Autodesk Inventor part; units mm, degrees
(part 2 of 2)
  spline S168 degree 2 poles (30.2962, -217.2786) (29.7923, -217.2786) (29.3205, -216.4956) (29.3205, -215.6929) knots 0 0 0 1 2 2 2
  spline S169 degree 2 poles (29.3205, -215.6929) (29.3205, -214.8679) (29.7972, -214.1047) (30.2962, -214.1047) knots 0 0 0 1 2 2 2
  spline S170 degree 2 poles (30.2962, -214.1047) (30.7976, -214.1047) (31.2693, -214.8951) (31.2693, -215.6904) knots 0 0 0 1 2 2 2
  spline S171 degree 2 poles (30.7457, -216.6191) (30.805, -216.4685) (30.8544, -216.0041) (30.8544, -215.6904) knots 0 0 0 1 2 2 2
  spline S172 degree 2 poles (30.8544, -215.6904) (30.8544, -215.3767) (30.805, -214.9148) (30.7432, -214.7592) knots 0 0 0 1 2 2 2
  spline S173 degree 2 poles (30.7432, -214.7592) (30.6815, -214.6036) (30.4666, -214.4431) (30.2962, -214.4431) knots 0 0 0 1 2 2 2
  spline S174 degree 2 poles (30.2962, -214.4431) (30.1257, -214.4431) (29.9059, -214.6036) (29.8417, -214.7642) knots 0 0 0 1 2 2 2
  spline S175 degree 2 poles (29.8417, -214.7642) (29.7799, -214.9198) (29.7355, -215.394) (29.7355, -215.6929) knots 0 0 0 1 2 2 2
  spline S176 degree 2 poles (29.7355, -215.6929) (29.7355, -216.014) (29.775, -216.4438) (29.8392, -216.6117) knots 0 0 0 1 2 2 2
  spline S177 degree 2 poles (29.8392, -216.6117) (29.8985, -216.7698) (30.1183, -216.9402) (30.2962, -216.9402) knots 0 0 0 1 2 2 2
  spline S178 degree 2 poles (30.2962, -216.9402) (30.4641, -216.9402) (30.684, -216.7797) (30.7457, -216.6191) knots 0 0 0 1 2 2 2
  line L158 (33.5393, -217.2144) -> (31.6596, -217.2144)
  line L159 (31.6596, -217.2144) -> (31.6596, -216.7822)
  spline S179 degree 2 poles (31.6596, -216.7822) (31.8622, -216.592) (32.2228, -216.2388) (32.3957, -216.0486) knots 0 0 0 1 2 2 2
  spline S180 degree 2 poles (32.3957, -216.0486) (32.7439, -215.6657) (32.9984, -215.2063) (32.9984, -214.9618) knots 0 0 0 1 2 2 2
  spline S181 degree 2 poles (32.9984, -214.9618) (32.9984, -214.8333) (32.9193, -214.6407) (32.8477, -214.5789) knots 0 0 0 1 2 2 2
  spline S182 degree 2 poles (32.8477, -214.5789) (32.7761, -214.5172) (32.5883, -214.4554) (32.4747, -214.4554) knots 0 0 0 1 2 2 2
  spline S183 degree 2 poles (32.4747, -214.4554) (32.366, -214.4554) (32.1437, -214.5097) (32.0425, -214.5517) knots 0 0 0 1 2 2 2
  spline S184 degree 2 poles (32.0425, -214.5517) (31.956, -214.5863) (31.7955, -214.6851) (31.7461, -214.7197) knots 0 0 0 1 2 2 2
  line L160 (31.7461, -214.7197) -> (31.7238, -214.7197)
  line L161 (31.7238, -214.7197) -> (31.7238, -214.285)
  spline S185 degree 2 poles (31.7238, -214.285) (31.8498, -214.2232) (32.3018, -214.1022) (32.5044, -214.1022) knots 0 0 0 1 2 2 2
  spline S186 degree 2 poles (32.5044, -214.1022) (32.9317, -214.1022) (33.4133, -214.5542) (33.4133, -214.9395) knots 0 0 0 1 2 2 2
  spline S187 degree 2 poles (33.4133, -214.9395) (33.4133, -215.1198) (33.3293, -215.4212) (33.2552, -215.5496) knots 0 0 0 1 2 2 2
  spline S188 degree 2 poles (33.2552, -215.5496) (33.1811, -215.683) (32.9663, -215.9448) (32.8477, -216.0708) knots 0 0 0 1 2 2 2
  spline S189 degree 2 poles (32.8477, -216.0708) (32.655, -216.2807) (32.1833, -216.7303) (32.0425, -216.8612) knots 0 0 0 1 2 2 2
  line L162 (32.0425, -216.8612) -> (33.5393, -216.8612)
  line L163 (33.5393, -216.8612) -> (33.5393, -217.2144)
  spline S190 degree 2 poles (35.8735, -216.2264) (35.8735, -216.4611) (35.7178, -216.8587) (35.5869, -216.9921) knots 0 0 0 1 2 2 2
  spline S191 degree 2 poles (35.5869, -216.9921) (35.4511, -217.1329) (35.1102, -217.2786) (34.9052, -217.2786) knots 0 0 0 1 2 2 2
  spline S192 degree 2 poles (34.9052, -217.2786) (34.7002, -217.2786) (34.3618, -217.1403) (34.2334, -217.002) knots 0 0 0 1 2 2 2
  spline S193 degree 2 poles (34.2334, -217.002) (34.0753, -216.8365) (33.8974, -216.2807) (33.8974, -215.8757) knots 0 0 0 1 2 2 2
  spline S194 degree 2 poles (33.8974, -215.8757) (33.8974, -215.478) (34.0605, -214.8383) (34.2309, -214.6011) knots 0 0 0 1 2 2 2
  spline S195 degree 2 poles (34.2309, -214.6011) (34.3964, -214.369) (34.92, -214.1096) (35.2634, -214.1096) knots 0 0 0 1 2 2 2
  spline S196 degree 2 poles (35.2634, -214.1096) (35.3646, -214.1096) (35.5425, -214.1294) (35.6092, -214.1516) knots 0 0 0 1 2 2 2
  line L164 (35.6092, -214.1516) -> (35.6092, -214.5443)
  line L165 (35.6092, -214.5443) -> (35.5919, -214.5443)
  spline S197 degree 2 poles (35.5919, -214.5443) (35.5351, -214.5147) (35.3276, -214.4628) (35.209, -214.4628) knots 0 0 0 1 2 2 2
  spline S198 degree 2 poles (35.209, -214.4628) (34.8286, -214.4628) (34.3618, -214.9766) (34.3173, -215.4805) knots 0 0 0 1 2 2 2
  spline S199 degree 2 poles (34.3173, -215.4805) (34.4631, -215.3792) (34.7694, -215.268) (34.9521, -215.268) knots 0 0 0 1 2 2 2
  spline S200 degree 2 poles (34.9521, -215.268) (35.13, -215.268) (35.3967, -215.3397) (35.5425, -215.4484) knots 0 0 0 1 2 2 2
  spline S201 degree 2 poles (35.5425, -215.4484) (35.7104, -215.5743) (35.8735, -215.9646) (35.8735, -216.2264) knots 0 0 0 1 2 2 2
  spline S202 degree 2 poles (35.4585, -216.2437) (35.4585, -216.056) (35.3597, -215.8016) (35.251, -215.7126) knots 0 0 0 1 2 2 2
  spline S203 degree 2 poles (35.251, -215.7126) (35.1695, -215.6484) (34.967, -215.6064) (34.8608, -215.6064) knots 0 0 0 1 2 2 2
  spline S204 degree 2 poles (34.8608, -215.6064) (34.7175, -215.6064) (34.4483, -215.6929) (34.3173, -215.7744) knots 0 0 0 1 2 2 2
  spline S205 degree 2 poles (34.3173, -215.7744) (34.3149, -215.8189) (34.3099, -215.9028) (34.3099, -215.9671) knots 0 0 0 1 2 2 2
  spline S206 degree 2 poles (34.3099, -215.9671) (34.3099, -216.2832) (34.4334, -216.671) (34.5273, -216.7723) knots 0 0 0 1 2 2 2
  spline S207 degree 2 poles (34.5273, -216.7723) (34.6138, -216.8686) (34.8015, -216.9452) (34.9077, -216.9452) knots 0 0 0 1 2 2 2
  spline S208 degree 2 poles (34.9077, -216.9452) (35.1547, -216.9452) (35.4585, -216.5944) (35.4585, -216.2437) knots 0 0 0 1 2 2 2
  point P0 (0, 0)
  constraints: 2 other
emboss "Emboss1" sketch "Sketch14" operation cut depth 2.54 direction (-1, 0, 0)
sketch "Sketch16" plane through (5.08, 0, 0) normal (1, 0, 0) x (0, 0, -1)
  line L0 (-41.7074, -88.6682) -> (39.5726, -88.6682)
  line L1 (39.5726, -88.6682) -> (39.5726, -92.4782)
  line L2 (39.5726, -92.4782) -> (-41.7074, -92.4782)
  line L3 (-41.7074, -92.4782) -> (-41.7074, -88.6682)
  line L4 (22.7938, -210.0802) -> (-43.6417, -210.0802) projected
  line L5 (38.9083, -223.7962) -> (-43.6417, -223.7962) projected
  point P0 (0, 0)
  dimension "d195" = 3.81
  dimension "d692" = 135.128
  constraints: 8 end point, 2 parallel, 1 horizontal, 1 perpendicular
  measures "d195" distance between parallel lines of L0 L2
  measures "d692" distance between parallel lines of L5 L0
extrude "Extrusion13" add sketch "Sketch16" along normal blind 5.08
sketch "Sketch17" plane through (22.86, 33.2264, 21.4167) normal (0, 1, 0) x (1, 0, 0)
  line L0 (-6.858, 38.1) -> (0, 38.1) projected
  line L1 (-0.0061, 38.1) -> (0.0392, 38.1)
  line L2 (0, 65.5066) -> (0, -27.4066) projected
  line L3 (0, 35.5801) -> (0, 35.5243)
  line L4 (5, -24.2316) -> (5, 62.3316) projected
  line L5 (0, 38.1) -> (5, 38.1)
  line L6 (5, 38.1) -> (5, 0)
  line L7 (5, 0) -> (0, 0)
  line L8 (0, 0) -> (0, 38.1)
  point P0 (-22.86, 21.4167)
  point P1 (5, -23.8506)
  point P2 (5, 69.0626)
  point P3 (0, 0)
  point P4 (5, 38.1)
  point P5 (0, 38.1)
  point P6 (2.5, 0)
  point P7 (2.5, 38.1)
  dimension "d689" = 38.1
  constraints: 12 end point, 4 point on line, 2 horizontal, 2 midpoint, 2 parallel, 1 perpendicular
  measures "d689" distance of point (2.5, 0) point (2.5, 38.1)
extrude "Extrusion14" cut sketch "Sketch17" against normal blind 2.0066
sketch "Sketch18" plane through (0, 0, 0) normal (-1, 0, 0) x (0, 0, 1)
  arc A0 (46.2144, 33.1755) -> (48.7724, 30.6175) centre (48.0867, 32.4898) ccw projected
  circle A1 centre (48.0867, 32.4898) radius 4.5085
  arc A2 (-41.481, 33.1755) -> (-44.039, 30.6175) centre (-43.3533, 32.4898) ccw projected
  circle A3 centre (-43.3533, 32.4898) radius 4.5085
  arc A4 (-44.039, -223.194) -> (-41.481, -225.752) centre (-43.3533, -225.0662) ccw projected
  circle A5 centre (-43.3533, -225.0662) radius 4.5085
  arc A6 (46.2144, -225.752) -> (48.7724, -223.194) centre (48.0867, -225.0662) ccw projected
  circle A7 centre (48.0867, -225.0662) radius 4.5085
  point P0 (0, 0)
  dimension "d209" = 9.017
  dimension "d210" = 9.017
  dimension "d211" = 9.017
  dimension "d212" = 9.017
  constraints: 4 centre point, 4 coincident
  measures "d209" diameter of A1
  measures "d210" diameter of A3
  measures "d211" diameter of A5
  measures "d212" diameter of A7
extrude "Extrusion15" [suppressed]
sketch "Sketch19" plane through (22.86, -64.2842, -44.0899) normal (0, 0, -1) x (-1, 0, 0)
  line L0 (6.35, 0) -> (0, 0) projected
  line L1 (-5, 92.329) -> (-5, -156.337) projected
  line L2 (0, 0) -> (-5, 0)
  line L3 (-5, 0) -> (-5, 8.001)
  line L4 (-5, 8.001) -> (0, 8.001)
  line L5 (0, 8.001) -> (0, 0)
  point P0 (22.86, 64.2842)
  dimension "d216" = 5
  dimension "d219" = 8.001
  constraints: 8 end point, 2 parallel, 1 horizontal, 1 perpendicular, 1 point on line
  measures "d216" distance between parallel lines of L1 L5
  measures "d219" distance between parallel lines of L2 L4
extrude "Extrusion16" cut sketch "Sketch19" against normal blind 24.13
sketch "Sketch20" plane through (0, 0, 0) normal (-1, 0, 0) x (0, 0, 1)
  line L0 (-45.1249, 28.9592) -> (-41.5943, 28.9592)
  line L1 (-45.1249, 36.0204) -> (-41.5943, 36.0204)
  line L2 (-45.1249, 28.9592) -> (-47.1633, 32.4898)
  line L3 (-45.1249, 36.0204) -> (-47.1633, 32.4898)
  line L4 (-41.5943, 28.9592) -> (-39.5559, 32.4898)
  line L5 (-41.5943, 36.0204) -> (-39.5559, 32.4898)
  line L6 (49.8457, 36.0204) -> (51.8841, 32.4898)
  line L7 (49.8457, 28.9592) -> (51.8841, 32.4898)
  line L8 (46.3151, 28.9592) -> (49.8457, 28.9592)
  line L9 (46.3151, 36.0204) -> (49.8457, 36.0204)
  line L10 (46.3151, 36.0204) -> (44.2767, 32.4898)
  line L11 (46.3151, 28.9592) -> (44.2767, 32.4898)
  line L12 (-41.5943, -210.3596) -> (-39.5559, -213.8902)
  line L13 (-41.5943, -217.4208) -> (-39.5559, -213.8902)
  line L14 (-45.1249, -217.4208) -> (-41.5943, -217.4208)
  line L15 (-45.1249, -210.3596) -> (-41.5943, -210.3596)
  line L16 (-45.1249, -210.3596) -> (-47.1633, -213.8902)
  line L17 (-45.1249, -217.4208) -> (-47.1633, -213.8902)
  line L18 (49.8457, -210.3596) -> (51.8841, -213.8902)
  line L19 (49.8457, -217.4208) -> (51.8841, -213.8902)
  line L20 (46.3151, -217.4208) -> (49.8457, -217.4208)
  line L21 (46.3151, -210.3596) -> (49.8457, -210.3596)
  line L22 (46.3151, -210.3596) -> (44.2767, -213.8902)
  line L23 (46.3151, -217.4208) -> (44.2767, -213.8902)
  line L24 (43.6417, 31.2198) -> (-38.9083, 31.2198) projected
  line L25 (-45.2583, 37.5698) -> (49.9917, 37.5698) projected
  line L26 (53.1667, 34.3948) -> (53.1667, -226.9712) projected
  line L27 (41.2351, -73.1996) -> (44.7657, -73.1996)
  line L28 (44.7657, -73.1996) -> (46.8041, -76.7302)
  line L29 (41.2351, -73.1996) -> (39.1967, -76.7302)
  line L30 (44.7657, -80.2608) -> (46.8041, -76.7302)
  line L31 (41.2351, -80.2608) -> (39.1967, -76.7302)
  line L32 (41.2351, -80.2608) -> (44.7657, -80.2608)
  line L33 (-40.0449, -73.1996) -> (-42.0833, -76.7302)
  line L34 (-40.0449, -80.2608) -> (-42.0833, -76.7302)
  line L35 (-40.0449, -73.1996) -> (-36.5143, -73.1996)
  line L36 (-40.0449, -80.2608) -> (-36.5143, -80.2608)
  line L37 (-36.5143, -73.1996) -> (-34.4759, -76.7302)
  line L38 (-36.5143, -80.2608) -> (-34.4759, -76.7302)
  line L39 (-48.4333, -226.9712) -> (-48.4333, 34.3948) projected
  point P0 (0, 0)
  point P1 (-43.3596, 28.9592)
  point P2 (-43.3533, 32.4898)
  point P3 (48.0804, 28.9592)
  point P4 (-43.3596, -217.4208)
  point P5 (48.0804, -217.4208)
  point P6 (-16.6833, 31.2198)
  point P7 (43.0004, -80.2608)
  point P8 (-38.2796, -80.2608)
  dimension "d366" = 7.0612
  dimension "d367" = 120
  dimension "d368" = 120
  dimension "d369" = 120
  dimension "d370" = 120
  dimension "d371" = 3.5306
  dimension "d372" = 3.5306
  dimension "d373" = 3.5306
  dimension "d374" = 3.5306
  dimension "d375" = 3.5306
  dimension "d376" = 3.5306
  dimension "d377" = 0
  dimension "d378" = 7.6074
  dimension "d383" = 7.0612
  dimension "d384" = 120
  dimension "d385" = 120
  dimension "d386" = 120
  dimension "d387" = 120
  dimension "d388" = 3.5306
  dimension "d389" = 3.5306
  dimension "d390" = 3.5306
  dimension "d391" = 3.5306
  dimension "d392" = 3.5306
  dimension "d393" = 3.5306
  dimension "d394" = 0
  dimension "d395" = 7.6074
  dimension "d402" = 7.0612
  dimension "d403" = 120
  dimension "d404" = 120
  dimension "d405" = 120
  dimension "d406" = 120
  dimension "d407" = 3.5306
  dimension "d408" = 3.5306
  dimension "d409" = 3.5306
  dimension "d410" = 3.5306
  dimension "d411" = 3.5306
  dimension "d412" = 3.5306
  dimension "d413" = 0
  dimension "d414" = 7.6074
  dimension "d421" = 7.0612
  dimension "d422" = 120
  dimension "d423" = 120
  dimension "d424" = 120
  dimension "d425" = 120
  dimension "d426" = 3.5306
  dimension "d427" = 3.5306
  dimension "d428" = 3.5306
  dimension "d429" = 3.5306
  dimension "d430" = 3.5306
  dimension "d431" = 3.5306
  dimension "d432" = 0
  dimension "d433" = 7.6074
  dimension "d731" = 7.0612
  dimension "d732" = 120
  dimension "d733" = 120
  dimension "d734" = 120
  dimension "d735" = 120
  dimension "d736" = 3.5306
  dimension "d737" = 3.5306
  dimension "d738" = 3.5306
  dimension "d739" = 3.5306
  dimension "d740" = 3.5306
  dimension "d741" = 3.5306
  dimension "d742" = 0
  constraints: 72 end point, 12 horizontal, 6 midpoint
  measures "d366" distance from line of point (-43.36, 28.959) L1
  measures "d367" angle of L0 L2
  measures "d368" angle of L1 L3
  measures "d369" angle of L4 L0
  measures "d370" angle of L5 L1
  measures "d371" distance of L0.start L4.start
  measures "d372" distance of L1.start L5.start
  measures "d373" vertical distance of L1.start L3.end
  measures "d374" vertical distance of L0.start L2.end
  measures "d375" vertical distance of L5.start L5.end
  measures "d376" vertical distance of L4.start L4.end
  measures "d377" horizontal distance of L0.start L1.start
  measures "d378" distance of L4.end L2.end
  measures "d383" distance from line of point (48.08, 28.959) L9
  measures "d384" angle of L8 L11
  measures "d385" angle of L9 L10
  measures "d386" angle of L7 L8
  measures "d387" angle of L6 L9
  measures "d388" distance of L8.start L7.start
  measures "d389" distance of L9.start L6.start
  measures "d390" vertical distance of L9.start L10.end
  measures "d391" vertical distance of L8.start L11.end
  measures "d392" vertical distance of L6.start L6.end
  measures "d393" vertical distance of L7.start L7.end
  measures "d394" horizontal distance of L8.start L9.start
  measures "d395" distance of L7.end L11.end
  measures "d402" distance from line of point (-43.36, -217.421) L15
  measures "d403" angle of L14 L17
  measures "d404" angle of L15 L16
  measures "d405" angle of L13 L14
  measures "d406" angle of L12 L15
  measures "d407" distance of L14.start L13.start
  measures "d408" distance of L15.start L12.start
  measures "d409" vertical distance of L15.start L16.end
  measures "d410" vertical distance of L14.start L17.end
  measures "d411" vertical distance of L12.start L12.end
  measures "d412" vertical distance of L13.start L13.end
  measures "d413" horizontal distance of L14.start L15.start
  measures "d414" distance of L13.end L17.end
  measures "d421" distance from line of point (48.08, -217.421) L21
  measures "d422" angle of L20 L23
  measures "d423" angle of L21 L22
  measures "d424" angle of L19 L20
  measures "d425" angle of L18 L21
  measures "d426" distance of L20.start L19.start
  measures "d427" distance of L21.start L18.start
  measures "d428" vertical distance of L21.start L22.end
  measures "d429" vertical distance of L20.start L23.end
  measures "d430" vertical distance of L18.start L18.end
  measures "d431" vertical distance of L19.start L19.end
  measures "d432" horizontal distance of L20.start L21.start
  measures "d433" distance of L19.end L23.end
  measures "d731" distance from line of point (43, -80.261) L27
  measures "d732" angle of L32 L31
  measures "d733" angle of L27 L29
  measures "d734" angle of L30 L32
  measures "d735" angle of L28 L27
  measures "d736" distance of L31.start L32.end
  measures "d737" distance of L29.start L27.end
  measures "d738" vertical distance of L29.start L29.end
  measures "d739" vertical distance of L31.start L31.end
  measures "d740" vertical distance of L27.end L28.end
  measures "d741" vertical distance of L32.end L30.end
  measures "d742" horizontal distance of L31.start L29.start
extrude "Extrusion18" cut sketch "Sketch20" against normal blind 4
sketch "Sketch21" plane through (5.08, 0, 0) normal (1, 0, 0) x (0, 0, -1)
  line L0 (-46.8167, -220.6212) -> (-46.8167, 28.0448) projected
  line L1 (35.2253, -82.5002) -> (35.2253, -72.3775)
  line L2 (42.0833, -65.4455) -> (42.0833, -88.8822)
  circle A0 centre (38.2733, -76.7302) radius 1.9939
  line L3 (42.0833, -69.6717) -> (42.0833, -83.8957)
  line L4 (35.2282, -81.9518) -> (35.2282, -71.6157)
  line L5 (36.9596, -68.7879) -> (40.1092, -67.18)
  line L6 (41.4701, -65.8406) -> (42.0833, -64.6853)
  line L7 (36.9596, -84.7796) -> (40.1092, -86.3875)
  line L8 (41.4701, -87.7269) -> (42.0833, -88.8822)
  arc A1 (36.9596, -68.7879) -> (35.2282, -71.6157) centre (38.4032, -71.6157) ccw
  arc A2 (40.1092, -67.18) -> (41.4701, -65.8406) centre (38.6656, -64.3522) ccw
  arc A3 (35.2282, -81.9518) -> (36.9596, -84.7796) centre (38.4032, -81.9518) ccw
  arc A4 (41.4701, -87.7269) -> (40.1092, -86.3875) centre (38.6656, -89.2153) ccw
  circle A5 centre (38.2733, -76.7302) radius 1.9939 projected
  line L9 (44.0899, -222.6278) -> (44.0899, -64.2842) projected
  line L10 (42.0833, -65.4455) -> (42.0833, -64.6853)
  line L11 (-46.8167, -83.8422) -> (-46.8167, -69.6182)
  line L12 (-39.9587, -71.5622) -> (-39.9587, -81.8983)
  circle A6 centre (-43.0067, -76.7302) radius 1.9939 projected
  line L13 (-41.6901, -84.7261) -> (-44.8397, -86.334)
  line L14 (-46.1908, -87.655) -> (-46.8167, -88.8159)
  line L15 (-41.6901, -68.7344) -> (-44.8397, -67.1265)
  line L16 (-46.2239, -65.7423) -> (-46.8167, -64.5811)
  arc A7 (-44.8397, -86.334) -> (-46.1908, -87.655) centre (-43.3961, -89.1618) ccw
  arc A8 (-41.6901, -84.7261) -> (-39.9587, -81.8983) centre (-43.1337, -81.8983) ccw
  arc A9 (-39.9587, -71.5622) -> (-41.6901, -68.7344) centre (-43.1337, -71.5622) ccw
  arc A10 (-46.2239, -65.7423) -> (-44.8397, -67.1265) centre (-43.3961, -64.2987) ccw
  line L17 (-46.8167, -64.5811) -> (-46.8167, -88.8159)
  point P0 (0, 0)
  point P1 (41.0008, -66.7248)
  point P2 (41.0008, -86.8426)
  point P3 (-45.7211, -86.7839)
  point P4 (-45.7561, -66.6587)
  dimension "d766" = 6.858
  dimension "d767" = 3.9878
  dimension "d768" = 2.0396
  dimension "d769" = 2.0396
  dimension "d770" = 117.044
  dimension "d771" = 117.044
  dimension "d772" = 3.175
  dimension "d773" = 3.1496
  dimension "d774" = 3.1496
  dimension "d775" = 145
  dimension "d776" = 145
  dimension "d778" = 0
  dimension "d779" = 0
  dimension "d782" = 0
  dimension "d785" = 6.858
  dimension "d786" = 117.044
  dimension "d787" = 117.044
  dimension "d792" = 2.032
  dimension "d793" = 3.175
  dimension "d794" = 3.1496
  dimension "d795" = 3.1496
  constraints: 32 end point, 16 point on circle, 16 tangent, 12 point on line, 9 centre point, 6 equal radius, 2 parallel, 2 vertical, 1 coincident, 1 perpendicular
  measures "d766" distance between parallel lines of L2 L1
  measures "d767" diameter of A0
  measures "d768" vertical distance of point (41.001, -86.843) L8.end
  measures "d769" vertical distance of point (41.001, -66.725) L6.end
  measures "d770" angle of L5 L4
  measures "d771" angle of L4 L7
  measures "d772" radius of A1
  measures "d773" horizontal distance of L7.start L7.end
  measures "d774" horizontal distance of L5.start L5.end
  measures "d775" angle of L7 L8
  measures "d776" angle of L5 L6
  measures "d778" distance of A5.centre A0.centre
  measures "d779" distance of L8.end L2.end
  measures "d782" distance of A5.centre A0.centre
  measures "d785" distance between parallel lines of L0 L12
  measures "d786" angle of L13 L12
  measures "d787" angle of L15 L12
  measures "d792" vertical distance of point (-45.721, -86.784) L14.end
  measures "d793" radius of A7
  measures "d794" horizontal distance of L13.start L13.end
  measures "d795" horizontal distance of L15.start L15.end
extrude "Extrusion19" add sketch "Sketch21" along normal blind 22.86
sketch "Sketch22" plane through (16.08, -230.1462, -3.2973) normal (0, -1, 0) x (1, 0, 0)
  circle A0 centre (2.2292, -12.1283) radius 2.032
  line L0 (-16.08, -45.136) -> (6.78, -45.136) projected
  circle A1 centre (8.732, -12.1283) radius 2.032
  line L1 (11.78, 48.9456) -> (11.78, -37.6176) projected
  point P0 (-16.08, 3.2973)
  dimension "d445" = 4.064
  dimension "d446" = 33.0076
  dimension "d449" = 4.064
  dimension "d450" = 3.048
  constraints: 2 centre point
  measures "d445" diameter of A0
  measures "d446" distance from line of L0 A0.centre
  measures "d449" diameter of A1
  measures "d450" distance from line of L1 A1.centre
extrude "Extrusion20" cut sketch "Sketch22" against normal blind 6.35
fillet "Fillet6" radius 0.508 10 edges at (19.685, -64.2842, -48.4333) (19.685, -56.2842, -48.4333) (16.51, -60.2842, -48.4333) (15.748, -230.1462, 6.7027) (15.748, -230.1462, -3.2973) (19.431, 37.5698, -16.6833) (16.002, 37.5698, 2.3667) (19.431, 37.5698, 21.4167) (25.36, 33.2264, 21.4167) (25.36, -56.2832, -44.0899)
sketch "Sketch23" plane through (22.86, -225.8028, -3.2973) normal (0, -1, 0) x (1, 0, 0)
  line L0 (0, -37.6176) -> (0, 48.9456) projected
  line L1 (5, 48.9456) -> (5, -37.6176) projected
  line L2 (0, 10) -> (5, 10)
  line L3 (5, 10) -> (5, -0.0129)
  line L4 (5, -0.0129) -> (0, -0.0129)
  line L5 (0, -0.0129) -> (0, 10)
  point P0 (-22.86, 3.2973)
  constraints: 8 end point, 2 parallel, 1 horizontal, 1 perpendicular, 1 point on line
extrude "Extrusion21" cut sketch "Sketch23" against normal blind 6.35
sketch "Sketch24" plane through (8.636, -223.7962, -3.2973) normal (0, 1, 0) x (1, 0, 0)
  circle A0 centre (9.652, -31.572) radius 3.683
  line L0 (-3.556, 35.611) -> (-3.556, -46.939) projected
  point P0 (-8.636, -3.2973)
  point P1 (14.224, -56.464)
  dimension "d673" = 24.892
  dimension "d674" = 13.208
  dimension "d677" = 7.366
  constraints: 1 centre point
  measures "d673" vertical distance of point (14.224, -56.464) A0.centre
  measures "d674" distance from line of L0 A0.centre
  measures "d677" diameter of A0
extrude "Extrusion22" cut sketch "Sketch24" against normal blind 1.27
sketch "Sketch25" plane through (5.08, 0, 0) normal (1, 0, 0) x (0, 0, -1)
  line L0 (-46.8167, 4.2958) -> (23.2009, 4.2958)
  line L1 (14.3109, -8.4042) -> (-46.8167, -8.4042)
  line L2 (-46.8167, -8.4042) -> (-46.8167, 4.2958)
  circle A0 centre (-30.3067, -2.0542) radius 2 projected
  circle A1 centre (6.6909, -2.0542) radius 2 projected
  circle A2 centre (-11.8079, -2.0542) radius 2 projected
  line L3 (-46.8167, -220.6212) -> (-46.8167, 28.0448) projected
  line L4 (42.0833, 28.0448) -> (42.0833, -56.2832) projected
  line L5 (23.2009, 4.2958) -> (42.0833, 4.2958)
  line L6 (42.0833, 4.2958) -> (42.0833, -8.4042)
  line L7 (42.0833, -8.4042) -> (14.3109, -8.4042)
  point P0 (0, 0)
  point P1 (-11.8079, 4.2958)
  point P2 (-46.8167, -36.8286)
  point P3 (42.0833, -36.6918)
  dimension "d680" = 6.35
  dimension "d681" = 6.35
  dimension "d682" = 0
  dimension "d685" = 0
  dimension "d686" = 12.7
  constraints: 12 end point, 2 horizontal, 2 parallel, 1 midpoint, 1 perpendicular
  measures "d680" distance of point (-11.808, 4.296) A2.centre
  measures "d681" distance from line of L1 A2.centre
  measures "d682" distance between parallel lines of L3 L2
  measures "d685" distance between parallel lines of L4 L6
  measures "d686" distance between parallel lines of L7 L5
extrude "Extrusion23" add sketch "Sketch25" along normal blind 10.16
body "Solid1"
